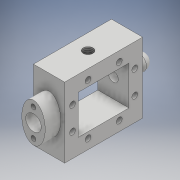
# Autodesk Inventor part: Steam Chest
Saved by Autodesk Inventor 2017 (Build 210142000, 142)
## iProperties
Created: 2018-11-18
Part Number: Steam Chest
Material: Generic
Document SubType Name: Modeling
Designer: Arman Grewal
Density: 1 g/cm^3
Appearance: Default
Author: Arman Grewal
Autodesk Inventor part; units mm, degrees
ref_plane "YZ Plane" through (0, 0, 0) normal (1, 0, 0) x (0, 1, 0)
ref_plane "XZ Plane" through (0, 0, 0) normal (0, 1, 0) x (-1, 0, 0)
ref_plane "XY Plane" through (0, 0, 0) normal (0, 0, 1) x (1, 0, 0)
sketch "Sketch1" plane through (0, 0, 0) normal (1, 0, 0) x (0, 1, 0)
  line L0 (20, 18) -> (-20, 18)
  line L1 (-20, 18) -> (-20, -18)
  line L2 (-20, -18) -> (20, -18)
  line L3 (20, -18) -> (20, 18)
  line L4 (13, -10) -> (-13, -10)
  line L5 (-13, -10) -> (-13, 10)
  line L6 (-13, 10) -> (13, 10)
  line L7 (13, 10) -> (13, -10)
  line L8 (20, 0) -> (-20, 0) construction
  line L9 (0, -18) -> (0, 18) construction
  circle A0 centre (16, 6) radius 1.5
  circle A1 centre (16, -6) radius 1.5
  circle A2 centre (-16, 6) radius 1.5
  circle A3 centre (-16, -6) radius 1.5
  circle A4 centre (8, 13) radius 1.5
  circle A5 centre (8, -13) radius 1.5
  circle A6 centre (-8, 13) radius 1.5
  circle A7 centre (-8, -13) radius 1.5
  point P0 (0, 0)
  dimension "d0" = 40
  dimension "d1" = 36
  dimension "d2" = 26
  dimension "d3" = 20
  dimension "d5" = 3
  dimension "d6" = 6
  dimension "d7" = 16
  dimension "d8" = 3
  dimension "d9" = 8
  dimension "d10" = 13
  dimension "d17" = 7
  dimension "d18" = 8
  dimension "d19" = 20
  dimension "d20" = 18
  constraints: 20 end point, 8 centre point, 6 symmetric about line, 4 midpoint, 4 parallel, 2 horizontal, 2 perpendicular, 6 other
  measures "d0" distance of L2.end L1.end
  measures "d1" distance of L1.end L0.end
  measures "d2" distance of L5.end L6.end
  measures "d3" distance of L4.end L5.end
  measures "d5" diameter of A0
  measures "d6" distance from line of L8 A0.centre
  measures "d7" distance from line of L9 A0.centre
  measures "d8" diameter of A4
  measures "d9" distance from line of L9 A4.centre
  measures "d10" distance from line of L8 A4.centre
  measures "d17" distance between parallel lines of L3 L7
  measures "d18" distance between parallel lines of L0 L6
  measures "d19" distance from line of point (0, 0) L3
  measures "d20" distance from line of point (0, 0) L0
extrude "Extrusion1" add sketch "Sketch1" along normal blind 16
sketch "Sketch2" plane through (0, -20, -18) normal (0, -1, 0) x (1, 0, 0)
  line L0 (0, 36) -> (16, 36) construction
  line L1 (8, 36) -> (8, 0) construction
  line L2 (0, 0) -> (16, 0) construction
  line L3 (16, 8) -> (16, 28) construction
  line L4 (16, 18) -> (0, 18) construction
  line L5 (8, 18) -> (8, 28) construction
  line L6 (8, 28) -> (8, 8) construction
  line L7 (8, 18) -> (14, 18) construction
  line L8 (14, 18) -> (2, 18) construction
  ellipse E0 centre (8, 18) end of major axis (14, 18) minor radius 10 construction
  ellipse E1 centre (8, 18) end of major axis (14, 18) minor radius 10
  dimension "d13" = 10
  dimension "d14" = 20
  dimension "d15" = 6
  dimension "d16" = 12
  constraints: 12 end point, 4 midpoint, 4 point on line, 3 horizontal, 2 coincident, 8 other
  measures "d13" distance of L5.start L5.end
  measures "d14" distance of L5.end L6.end
  measures "d15" distance of L5.start L7.end
  measures "d16" distance of L7.end L8.end
extrude "Extrusion2" add sketch "Sketch2" along normal blind 8
sketch "Sketch3" plane through (0, -28, -18) normal (0, -1, 0) x (1, 0, 0)
  ellipse E0 centre (8, 18) end of major axis (8, 28) minor radius 6 construction
  line L0 (8, 28) -> (8, 8) construction
  circle A0 centre (8, 25) radius 1.25
  circle A1 centre (8, 11) radius 1.25
  point P0 (0, 18)
  dimension "d23" = 2.5
  dimension "d24" = 7
  dimension "d25" = 2.5
  dimension "d26" = 7
  dimension "d27" = 0
  constraints: 2 centre point, 2 end point, 2 point on line, 1 vertical, 3 other
  measures "d23" diameter of A0
  measures "d24" distance of point (8, 18) A0.centre
  measures "d25" diameter of A1
  measures "d26" distance of point (8, 18) A1.centre
  measures "d27" distance from line of point (8, 18) L0
extrude "Extrusion3" cut sketch "Sketch3" against normal blind 6
thread "Thread1" size "M2.5x0.45" class "6H" standard "ANSI Metric M Profile" full length
thread "Thread2" size "M2.5x0.45" class "6H" standard "ANSI Metric M Profile" full length
sketch "Sketch4" plane through (0, -28, -18) normal (0, -1, 0) x (1, 0, 0)
  ellipse E0 centre (8, 18) end of major axis (8, 28) minor radius 6 construction
  line L0 (14, 18) -> (8, 18) construction
  circle A0 centre (8, 18) radius 2.5
  point P0 (0, 18)
  dimension "d34" = 5
  constraints: 2 end point, 1 centre point, 1 coincident, 1 horizontal, 1 horizontal alignment, 1 other
  measures "d34" diameter of A0
extrude "Extrusion4" cut sketch "Sketch4" against normal blind 90
sketch "Sketch5" plane through (0, -28, -18) normal (0, -1, 0) x (1, 0, 0)
  circle A0 centre (8, 18) radius 2.5 construction
  line L0 (5.5, 18) -> (8, 18) construction
  circle A1 centre (8, 18) radius 4
  point P0 (0, 18)
  dimension "d37" = 8
  constraints: 2 end point, 1 centre point, 1 coincident, 1 horizontal, 1 horizontal alignment, 1 other
  measures "d37" diameter of A1
extrude "Extrusion5" cut sketch "Sketch5" against normal blind 8
chamfer "Chamfer1" distance 1 angle 45 2 edges at (6.75, -22, 7) (6.75, -22, -7)
chamfer "Chamfer2" distance 1 angle 45 1 edges at (4, -20, 0)
sketch "Sketch6" plane through (0, -20, 18) normal (0, 0, 1) x (1, 0, 0)
  line L0 (0, 40) -> (16, 40) construction
  line L1 (8, 40) -> (8, 0) construction
  line L2 (0, 0) -> (16, 0) construction
  circle A0 centre (8, 20) radius 2.5 construction
  circle A1 centre (8, 20) radius 2.5
  point P0 (0, 20)
  dimension "d46" = 5
  constraints: 3 midpoint, 2 centre point, 2 end point, 1 coincident, 1 concentric
  measures "d46" diameter of A0
extrude "Extrusion6" cut sketch "Sketch6" against normal blind 6
sketch "Sketch7" plane through (8, 0, 12) normal (0, 0, 1) x (1, 0, 0)
  circle A0 centre (0, 0) radius 1.5
  line L0 (-8, -13) -> (8, -13) projected
  point P0 (-8, 0)
  dimension "d49" = 3
  dimension "d50" = 8
  dimension "d51" = 13
  constraints: 1 centre point
  measures "d49" diameter of A0
  measures "d50" distance of A0.centre point (-8, 0)
  measures "d51" distance from line of L0 A0.centre
extrude "Extrusion7" cut sketch "Sketch7" against normal blind 6
chamfer "Chamfer3" distance 1 angle 45 1 edges at (6.5, 0, 12)
thread "Thread3" size "M5x0.8" class "6H" standard "ANSI Metric M Profile" full length
sketch "Sketch8" plane through (0, 20, 18) normal (0, 1, 0) x (1, 0, 0)
  circle A0 centre (8, 18) radius 2.5 construction
  line L0 (5.5, 18) -> (8, 18) construction
  circle A1 centre (8, 18) radius 4
  point P0 (0, 18)
  dimension "d59" = 8
  constraints: 2 end point, 1 centre point, 1 coincident, 1 horizontal, 1 horizontal alignment, 1 other
  measures "d59" diameter of A1
extrude "Extrusion8" add sketch "Sketch8" along normal blind 10
fillet "Fillet1" radius 4 1 edges at (4, 30, 0)
fillet "Fillet2" radius 2 1 edges at (4, 20, 0)
sketch "Sketch9" plane through (0, 13, -10) normal (0, -1, 0) x (1, 0, 0)
  circle A0 centre (8, 10) radius 2.5 construction
  line L0 (5.5, 10) -> (8, 10) construction
  circle A1 centre (8, 10) radius 2.5
  point P0 (0, 10)
  constraints: 2 end point, 1 centre point, 1 coincident, 1 horizontal, 1 horizontal alignment, 2 other
extrude "Extrusion9" cut sketch "Sketch9" against normal blind 16
fillet "Fillet3" radius 2 1 edges at (5.5, 29, 0)
body "Solid1"
